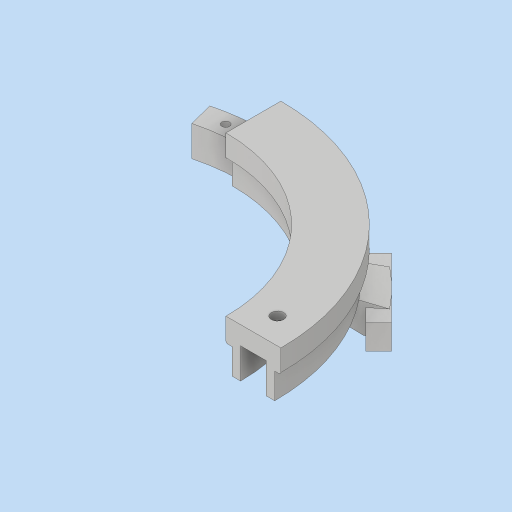
# Autodesk Inventor part: kolejnice
Saved by Autodesk Inventor 2024 (Build 280153000, 153)
## iProperties
Created: 2021-04-14
Part Number: kolejnice
Material: Generic
Document SubType Name: Modeling
Designer: Karbosch
Density: 1 g/cm^3
Appearance: Default
Mass: 414.582 g
Surface Area: 575.113 cm^2
Volume: 414.582 cm^3
Author: Karbosch
Autodesk Inventor part; units mm, degrees
sketch "Sketch1" plane through (0, 0, 0) normal (0, 1, 0) x (-1, 0, 0)
  circle A0 centre (0, 0) radius 130
  dimension "d3" = 260
  constraints: 1 centre point, 1 coincident
  measures "d3" diameter of A0
sketch "Sketch2" plane through (0, 0, 0) normal (1, 0, 0) x (0, 1, 0)
  line L0 (0, -130) -> (0, -175)
  line L1 (0, -175) -> (-19, -175)
  line L2 (-19, -175) -> (-19, -170)
  line L3 (-19, -170) -> (-40, -170)
  line L4 (-40, -170) -> (-40, -135)
  line L5 (-40, -135) -> (-19, -135)
  line L6 (-19, -135) -> (-19, -130)
  line L7 (-19, -130) -> (0, -130)
  line L8 (50.5, 0) -> (-78.5, 0)
  point P0 (0, 0)
  dimension "d4" = 45
  dimension "d5" = 19
  dimension "d7" = 5
  dimension "d8" = 35
  constraints: 18 end point, 5 perpendicular, 2 point on line, 2 vertical, 1 horizontal
  measures "d4" distance of L0.start L0.end
  measures "d5" distance of L0.end L1.end
  measures "d7" distance of L1.end L2.end
  measures "d8" distance of L3.end L4.end
revolve "Revolution1" add sketch "Sketch2" angle 90 about axis through (0, 50.5, 0) along (0, -1, 0)
sketch "Sketch5" plane through (130, 0, 0) normal (0, 0, 1) x (1, 0, 0)
  line L0 (5, -19) -> (5, -40) projected
  line L1 (5, -40) -> (40, -40) projected
  line L2 (12, -40) -> (12, -15)
  line L3 (12, -15) -> (33, -15)
  line L4 (33, -15) -> (33, -40)
  line L5 (12, -40) -> (33, -40)
  line L6 (-130, 8) -> (-130, -48) projected
  point P0 (-130, 0)
  dimension "d10" = 7
  dimension "d11" = 25
  dimension "d12" = 21
  constraints: 8 end point, 3 perpendicular, 2 point on line, 1 collinear
  measures "d10" distance of L0.end L2.start
  measures "d11" distance of L2.start L2.end
  measures "d12" distance of L2.end L3.end
revolve "Revolution2" cut sketch "Sketch5" angle 15 about axis through (0, 70.5, 0) along (0, 1, 0)
sketch "Sketch6" plane through (0, -40, -170) normal (-1, 0, 0) x (0, 0, 1)
  line L0 (170, 48) -> (170, -8) projected
  line L1 (0, 0) -> (170, 0) projected
  line L2 (7.3, 0) -> (27.7, 0)
  line L3 (27.7, 0) -> (27.7, 25)
  line L4 (27.7, 25) -> (7.3, 25)
  line L5 (7.3, 25) -> (7.3, 0)
  point P0 (170, 40)
  dimension "d57" = 20.4
  dimension "d58" = 25
  constraints: 8 end point, 2 parallel, 1 horizontal, 1 perpendicular, 1 point on line
  measures "d57" distance of L4.end L3.end
  measures "d58" distance of L3.end L2.end
revolve "Revolution3" add sketch "Sketch6" angle 14.5 about axis through (0, 70.5, 0) along (0, 1, 0)
ref_plane "Work Plane1" through (91.9239, 0, -91.9239) normal (-0.7071, 0, -0.7071) x (0, -1, 0)
sketch "Sketch7" plane through (91.9239, 0, -91.9239) normal (-0.7071, 0, -0.7071) x (0, -1, 0)
  line L0 (45, -57.85) -> (45, -42.85)
  line L1 (45, -42.85) -> (65, -42.85)
  line L2 (65, -42.85) -> (65, -57.85)
  line L3 (65, -57.85) -> (45, -57.85)
  line L4 (40, -40) -> (40, 9.7918) projected
  line L5 (40, -40) -> (45, -40)
  line L6 (45, -40) -> (45, -42.85)
  point P0 (0, 130)
  dimension "d22" = 15
  dimension "d23" = 20
  constraints: 12 end point, 4 perpendicular
  measures "d22" distance of L0.start L0.end
  measures "d23" distance of L0.end L1.end
extrude "Extrusion1" add sketch "Sketch7" along normal mid plane 70
sketch "Sketch9" plane through (97.4747, -65, -146.9721) normal (-0.7071, 0, 0.7071) x (0.7071, 0, 0.7071)
  line L0 (70, 0) -> (70, 20) projected
  line L1 (70, 10) -> (0, 10)
  line L2 (0, 20) -> (0, 0) projected
  line L3 (35, 10) -> (60, 10)
  line L4 (60, 10) -> (60, 18)
  line L5 (35, 10) -> (10, 10)
  line L6 (10, 10) -> (10, 2.5277)
  line L7 (55, 5) -> (65, 5)
  line L8 (65, 5) -> (65, 15)
  line L9 (65, 15) -> (55, 15)
  line L10 (55, 15) -> (55, 5)
  line L11 (55, 5) -> (65, 15) construction
  line L12 (65, 5) -> (55, 15) construction
  line L13 (5, 5) -> (15, 5)
  line L14 (15, 5) -> (15, 15)
  line L15 (15, 15) -> (5, 15)
  line L16 (5, 15) -> (5, 5)
  line L17 (5, 5) -> (15, 15) construction
  line L18 (15, 5) -> (5, 15) construction
  point P0 (35, 65)
  dimension "d28" = 25
  dimension "d29" = 25
  dimension "d31" = 10
  dimension "d32" = 10
  dimension "d33" = 10
  dimension "d34" = 10
  constraints: 34 end point, 7 midpoint, 4 parallel, 4 perpendicular, 2 horizontal, 2 point on line
  measures "d28" distance of L3.start L3.end
  measures "d29" distance of L3.start L5.end
  measures "d31" distance of L9.end L8.end
  measures "d32" distance of L8.end L7.end
  measures "d33" distance of L15.end L14.end
  measures "d34" distance of L14.end L13.end
sketch "Sketch10" plane through (97.4747, -65, -146.9721) normal (-0.7071, 0, 0.7071) x (0.7071, 0, 0.7071)
  line L0 (70, 10) -> (0, 10)
  line L1 (35, 10) -> (60, 10)
  line L2 (60, 10) -> (60, 18)
  line L3 (35, 10) -> (10, 10)
  line L4 (10, 10) -> (10, 2.5277)
  line L5 (55, 5) -> (65, 5)
  line L6 (65, 5) -> (65, 15)
  line L7 (65, 15) -> (55, 15)
  line L8 (55, 15) -> (55, 5)
  line L9 (55, 5) -> (65, 15) construction
  line L10 (65, 5) -> (55, 15) construction
  line L11 (5, 5) -> (15, 5)
  line L12 (15, 5) -> (15, 15)
  line L13 (15, 15) -> (5, 15)
  line L14 (5, 15) -> (5, 5)
  line L15 (5, 5) -> (15, 15) construction
  line L16 (15, 5) -> (5, 15) construction
  point P0 (35, 65)
  dimension "d35" = 25
  dimension "d36" = 25
  dimension "d37" = 10
  dimension "d38" = 10
  dimension "d39" = 10
  dimension "d40" = 10
  constraints: 34 end point, 5 midpoint, 4 parallel, 4 perpendicular, 2 horizontal, 2 point on line
  measures "d35" distance of L1.start L1.end
  measures "d36" distance of L1.start L3.end
  measures "d37" distance of L7.end L6.end
  measures "d38" distance of L6.end L5.end
  measures "d39" distance of L13.end L12.end
  measures "d40" distance of L12.end L11.end
hole "Hole1" at (104.5457, -55, -139.9011) at (139.9011, -55, -104.5457) direction (0.7071, 0, -0.7071) diameter 6.4 end through all
sketch "Sketch11" plane through (91.9239, 0, -91.9239) normal (-0.7071, 0, -0.7071) x (0, -1, 0)
  point P0 (0, 130)
sketch "Sketch12" plane through (91.9239, 0, -91.9239) normal (-0.7071, 0, -0.7071) x (0, -1, 0)
  line L0 (65, -42.85) -> (65, -57.85) projected
  line L1 (19, -40) -> (40, -40) projected
  line L2 (40, 14.7416) -> (40, -11.1621) projected
  line L3 (40, -5) -> (65, -42.85)
  line L4 (65, -42.85) -> (65, -50.35)
  line L5 (40, -5) -> (40, 34.5406) projected
  line L6 (40, -5) -> (40, -40)
  line L7 (65, -50.35) -> (45, -57.85)
  line L8 (45, -57.85) -> (40, -40)
  line L9 (-13, 130) -> (78, 130) projected
  point P0 (0, 130)
  constraints: 10 end point, 1 collinear, 1 midpoint, 1 point on line
revolve "Revolution4" add sketch "Sketch12" angle 12.91 mid plane about axis through (0, 70.5, 0) along (0, -1, 0)
sketch "Sketch13" plane through (0, 0, -130) normal (0, 1, 0) x (1, 0, 0)
  line L0 (0, -130) -> (161.4137, -107.3148)
  line L1 (0, -130) -> (163, -130)
  line L2 (-19.8043, 10.9151) -> (-22.6435, 31.1166)
  circle A0 centre (0, -130) radius 152.5
  line L3 (-21.2239, 21.0159) -> (-8.7133, 29.4565)
  line L4 (151.0159, -108.7761) -> (168.9314, -124.1402)
  point P0 (0, -130)
  dimension "d60" = 163
  dimension "d61" = 8
  constraints: 10 end point, 2 point on circle, 1 centre point, 1 coincident, 1 equal length, 1 horizontal, 1 midpoint, 1 point on line
  measures "d60" distance of L0.start L0.end
  measures "d61" angle of L1 L0
hole "Hole2" at (-21.2239, 0, -151.0159) at (151.0159, 0, -21.2239) direction (0, -1, 0) diameter 6.4 end through all counterbore diameter 10.2 counterbore depth 6.5
fillet "Fillet3" radius 1.5 2 edges at (91.9239, -19, -91.9239) (123.7437, -19, -123.7437)
sketch "Náčrt16" plane through (108.0813, -65, -157.5787) normal (0, -1, 0) x (0.7071, 0, -0.7071)
  point P0 (-187.85, 35)
sketch "Sketch18" plane through (108.0813, -65, -157.5787) normal (0, -1, 0) x (0.7071, 0, -0.7071)
  line L0 (0, 0) -> (-7.5, 0)
  line L1 (-7.5, 0) -> (-7.5, 10)
  line L2 (-7.5, 70) -> (-7.5, 60)
  line L3 (-9.95, 15.1) -> (-5.05, 15.1)
  line L4 (-5.05, 15.1) -> (-5.05, 4.9)
  line L5 (-5.05, 4.9) -> (-9.95, 4.9)
  line L6 (-9.95, 4.9) -> (-9.95, 15.1)
  line L7 (-9.95, 15.1) -> (-5.05, 4.9) construction
  line L8 (-5.05, 15.1) -> (-9.95, 4.9) construction
  line L9 (-9.95, 65.1) -> (-5.05, 65.1)
  line L10 (-5.05, 65.1) -> (-5.05, 54.9)
  line L11 (-5.05, 54.9) -> (-9.95, 54.9)
  line L12 (-9.95, 54.9) -> (-9.95, 65.1)
  line L13 (-9.95, 65.1) -> (-5.05, 54.9) construction
  line L14 (-5.05, 65.1) -> (-9.95, 54.9) construction
  point P0 (-187.85, 35)
  dimension "d86" = 7.5
  dimension "d87" = 10
  dimension "d88" = 10
  dimension "d104" = 4.9
  dimension "d105" = 10.2
  dimension "d106" = 4.9
  dimension "d107" = 10.2
  constraints: 30 end point, 4 midpoint, 4 parallel, 2 horizontal, 2 perpendicular, 1 vertical
  measures "d86" distance of L0.start L0.end
  measures "d87" distance of L0.end L1.end
  measures "d88" distance of L2.start L2.end
  measures "d104" distance of L4.end L5.end
  measures "d105" distance of L3.end L4.end
  measures "d106" distance of L10.end L11.end
  measures "d107" distance of L9.end L10.end
extrude "Extrusion5" cut sketch "Sketch18" against normal blind 15.1
ref_plane "Work Plane3" through (-21.2239, -285.2935, -151.0159) normal (0.9903, 0, -0.1392) x (0, 1, 0)
ref_plane "Work Plane5" through (-21.2239, -15, -151.0159) normal (0.0698, 0, 0.9976) x (0.9976, 0, -0.0698)
sketch "Sketch19" plane through (-21.2239, -15, -151.0159) normal (0.0698, 0, 0.9976) x (0.9976, 0, -0.0698)
  line L0 (5.1, -10) -> (-5.1, -10)
  line L1 (-5.1, -10) -> (-5.1, -14.9)
  line L2 (-5.1, -14.9) -> (5.1, -14.9)
  line L3 (5.1, -14.9) -> (5.1, -10)
  point P0 (10.6379, 15)
  dimension "d103" = 10.2
  constraints: 8 end point, 1 perpendicular, 1 vertical
  measures "d103" distance of L0.start L0.end
extrude "Extrusion6" cut sketch "Sketch19" against normal blind 15
sketch "Sketch20" plane through (-21.2239, -15, -151.0159) normal (-0.0698, 0, -0.9976) x (-0.9976, 0, 0.0698)
  line L0 (-5.1, -14.9) -> (-5.1, -10) projected
  line L1 (-5.1, -10) -> (5.1, -10)
  line L2 (5.1, -10) -> (5.1, -14.9)
  line L3 (5.1, -14.9) -> (-5.1, -14.9)
  line L4 (-5.1, -14.9) -> (-5.1, -10)
  point P0 (10.6379, 15)
  point P1 (5, -10)
  point P2 (5, -14.9)
  constraints: 8 end point, 1 parallel, 1 perpendicular, 1 vertical
extrude "Extrusion7" cut sketch "Sketch20" against normal blind 5.1
body "Solid1"
